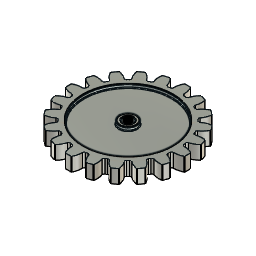
spur gear (Autodesk Fusion 360 design; units mm, degrees)
part number: 2025-09-15-00-14-42-283
Autodesk Fusion 360 part; units mm, degrees
sketch "Sketch1" plane through (0, 0, 0) normal (0, 0, 1) x (1, 0, 0)
  line L0 (0, 0) -> (0, 120) construction
  line L1 (0, 0) -> (120, 0) construction
  line L2 (7.5783, 72.1028) -> (12.464, 118.5873)
  line L3 (13.688, 86.4227) -> (18.0383, 113.8896)
  arc A0 (7.7182, 74.3498) -> (4.8497, 86.8626) centre (-18.7417, 74.8692) ccw
  arc A1 (4.0041, 87.4083) -> (-4.0041, 87.4083) centre (0, 0) ccw
  arc A2 (7.2846, 79.6676) -> (80, 0) centre (0, 0) ccw
  line L4 (11.3415, 71.6074) -> (0, 0)
  arc A3 (11.3415, 71.6074) -> (9.8771, 71.824) centre (0, 0) ccw
  arc A4 (7.7182, 74.3498) -> (9.8771, 71.824) centre (10.2177, 74.3007) ccw
  arc A5 (4.8497, 86.8626) -> (4.0041, 87.4083) centre (3.9583, 86.4094) ccw
  line L5 (-11.3415, 71.6074) -> (0, 0)
  arc A6 (-9.8771, 71.824) -> (-7.7182, 74.3498) centre (-10.2177, 74.3007) ccw
  arc A7 (-9.8771, 71.824) -> (-11.3415, 71.6074) centre (0, 0) ccw
  arc A8 (-4.8497, 86.8626) -> (-7.7182, 74.3498) centre (18.7417, 74.8692) ccw
  arc A9 (-4.0041, 87.4083) -> (-4.8497, 86.8626) centre (-3.9583, 86.4094) ccw
  arc A10 (-87.5, 0) -> (87.5, 0) centre (0, 0) ccw
  arc A11 (13.688, 86.4227) -> (-4.0041, 87.4083) centre (0, 0) ccw
  dimension "d1" = 160
  dimension "d2" = 175
  dimension "d3" = 145
  dimension "d5" = 6
  dimension "d6" = 9
  dimension "d7" = 2.5
  dimension "d8" = 1
  constraint coincident L0.start L1.start
  constraint concentric A1 A2
  constraint vertical L0
  constraint perpendicular L0 L1
  constraint tangent L2 A0
  constraint coincident L1 A10.end
  constraint coincident L1 A2.end
  constraint coincident A0 A2.start
  constraint coincident L2.start A3
  constraint coincident L2.start A0
  constraint tangent A3 A4
  constraint tangent A0 A4
  constraint tangent A0 A5
  constraint tangent A1 A5
  constraint symmetric L0 A0 A8
  constraint symmetric L0 A10.end A10.start
  constraint symmetric L0 A1 A10
  constraint symmetric L0 L4.start L5.start
  constraint symmetric L0 L1.start A1.centre
  constraint symmetric L0 A3 A7
  constraint symmetric L0 A3.end A6.start
  constraint symmetric L0 A0.start A6.end
  constraint symmetric L0 A4 A6
  constraint symmetric L0 A0.end A8.start
  constraint symmetric L0 A1.start A1.end
  constraint symmetric L0 A5 A9
  constraint concentric A10 A11
  measures "d1" diameter of A2
  measures "d2" diameter of A1
  measures "d3" diameter of A3
  measures "d5" angle of L0 L2
  measures "d6" angle of L0 L3
  measures "d7" radius of A4
  measures "d8" radius of A5
sketch "Sketch2" plane through (0, 0, 0) normal (0, 0, 1) x (1, 0, 0)
extrude "Extrude1" add sketch "Sketch1" along normal blind 20 contours A0 A2 L4 A3 A4 L5 A6 A7 A8 | A0 A1 A2 A5 A8 A9 A11 makes body 1
pattern_circular "C-Pattern1" count 20 over 360 about axis through (0, 0, 1.75) along (0, 0, 1) of bodies 1 makes body 2 at (-7.561, 47.7383, 6.6667) makes body 3 at (-28.1691, 38.7805, 0) makes body 4 at (-38.7742, 28.1777, 0) makes body 5 at (-45.5839, 14.8167, 0) makes body 6 at (-47.9315, 0.0054, 0) makes body 7 at (-45.5872, -14.8066, 0) makes body 8 at (-38.7805, -28.1691, 0) makes body 9 at (-28.1777, -38.7742, 0) makes body 10 at (-14.8167, -45.5839, 0) makes body 11 at (-0.0054, -47.9315, 0) makes body 12 at (14.8066, -45.5872, 0) makes body 13 at (28.1691, -38.7805, 0) makes body 14 at (38.7742, -28.1777, 0) makes body 15 at (45.5839, -14.8167, 0) makes body 16 at (47.9315, -0.0054, 0) makes body 17 at (45.5872, 14.8066, 0) makes body 18 at (38.7805, 28.1691, 0) makes body 19 at (28.1777, 38.7742, 0) makes body 20 at (7.561, 47.7383, 6.6667)
combine "Combine1" operation add target body 20 tool bodies 19 18 17 16 15 14 13 12 11 10 9 8 7 6 5 4 3 2 1
sketch "Sketch3" plane through (0, 0, 20) normal (0, 0, 1) x (-1, 0, 0)
  arc A0 (-30.3158, -68.3258) -> (-31.4544, -81.1126) centre (-5.3114, -76.9963) ccw
  arc A1 (-31.4544, -81.1126) -> (-30.8187, -81.8929) centre (-30.4665, -80.957) ccw
  arc A2 (-30.8187, -81.8929) -> (-23.2026, -84.3676) centre (0, 0) ccw
  arc A3 (-23.2026, -84.3676) -> (-22.2297, -84.1099) centre (-22.9374, -83.4034) ccw
  arc A4 (-22.2297, -84.1099) -> (-15.6349, -73.0959) centre (-40.9603, -65.4133) ccw
  arc A5 (-12.8011, -71.3609) -> (-15.6349, -73.0959) centre (-13.2426, -73.8216) ccw
  arc A6 (-12.8011, -71.3609) -> (-9.8771, -71.824) centre (0, 0) ccw
  arc A7 (-7.7182, -74.3498) -> (-9.8771, -71.824) centre (-10.2177, -74.3007) ccw
  arc A8 (-7.7182, -74.3498) -> (-4.8497, -86.8626) centre (18.7417, -74.8692) ccw
  arc A9 (-4.8497, -86.8626) -> (-4.0041, -87.4083) centre (-3.9583, -86.4094) ccw
  arc A10 (-4.0041, -87.4083) -> (4.0041, -87.4083) centre (0, 0) ccw
  arc A11 (4.0041, -87.4083) -> (4.8497, -86.8626) centre (3.9583, -86.4094) ccw
  arc A12 (4.8497, -86.8626) -> (7.7182, -74.3498) centre (-18.7417, -74.8692) ccw
  arc A13 (9.8771, -71.824) -> (7.7182, -74.3498) centre (10.2177, -74.3007) ccw
  arc A14 (9.8771, -71.824) -> (12.8011, -71.3609) centre (0, 0) ccw
  arc A15 (15.6349, -73.0959) -> (12.8011, -71.3609) centre (13.2426, -73.8216) ccw
  arc A16 (15.6349, -73.0959) -> (22.2297, -84.1099) centre (40.9603, -65.4133) ccw
  arc A17 (22.2297, -84.1099) -> (23.2026, -84.3676) centre (22.9374, -83.4034) ccw
  arc A18 (23.2026, -84.3676) -> (30.8187, -81.8929) centre (0, 0) ccw
  arc A19 (30.8187, -81.8929) -> (31.4544, -81.1126) centre (30.4665, -80.957) ccw
  arc A20 (31.4544, -81.1126) -> (30.3158, -68.3258) centre (5.3114, -76.9963) ccw
  arc A21 (31.5886, -65.2565) -> (30.3158, -68.3258) centre (32.6778, -67.5067) ccw
  arc A22 (31.5886, -65.2565) -> (34.2264, -63.9125) centre (0, 0) ccw
  arc A23 (37.4576, -64.6869) -> (34.2264, -63.9125) centre (35.4066, -66.1164) ccw
  arc A24 (37.4576, -64.6869) -> (47.133, -73.1239) centre (59.1694, -49.5543) ccw
  arc A25 (47.133, -73.1239) -> (48.138, -73.0684) centre (47.5878, -72.2333) ccw
  arc A26 (48.138, -73.0684) -> (54.6167, -68.3613) centre (0, 0) ccw
  arc A27 (54.6167, -68.3613) -> (54.98, -67.4227) centre (53.9925, -67.58) ccw
  arc A28 (54.98, -67.4227) -> (49.9459, -55.6136) centre (28.8446, -71.5866) ccw
  arc A29 (50.2079, -52.3012) -> (49.9459, -55.6136) centre (51.9392, -54.1047) ccw
  arc A30 (50.2079, -52.3012) -> (52.3012, -50.2079) centre (0, 0) ccw
  arc A31 (55.6136, -49.9459) -> (52.3012, -50.2079) centre (54.1047, -51.9392) ccw
  arc A32 (55.6136, -49.9459) -> (67.4227, -54.98) centre (71.5866, -28.8446) ccw
  arc A33 (67.4227, -54.98) -> (68.3613, -54.6167) centre (67.58, -53.9925) ccw
  arc A34 (68.3613, -54.6167) -> (73.0684, -48.138) centre (0, 0) ccw
  arc A35 (73.0684, -48.138) -> (73.1239, -47.133) centre (72.2333, -47.5878) ccw
  arc A36 (73.1239, -47.133) -> (64.6869, -37.4576) centre (49.5543, -59.1694) ccw
  arc A37 (63.9125, -34.2264) -> (64.6869, -37.4576) centre (66.1164, -35.4066) ccw
  arc A38 (63.9125, -34.2264) -> (65.2565, -31.5886) centre (0, 0) ccw
  arc A39 (68.3258, -30.3158) -> (65.2565, -31.5886) centre (67.5067, -32.6778) ccw
  arc A40 (68.3258, -30.3158) -> (81.1126, -31.4544) centre (76.9963, -5.3114) ccw
  arc A41 (81.1126, -31.4544) -> (81.8929, -30.8187) centre (80.957, -30.4665) ccw
  arc A42 (81.8929, -30.8187) -> (84.3676, -23.2026) centre (0, 0) ccw
  arc A43 (84.3676, -23.2026) -> (84.1099, -22.2297) centre (83.4034, -22.9374) ccw
  arc A44 (84.1099, -22.2297) -> (73.0959, -15.6349) centre (65.4133, -40.9603) ccw
  arc A45 (71.3609, -12.8011) -> (73.0959, -15.6349) centre (73.8216, -13.2426) ccw
  arc A46 (71.3609, -12.8011) -> (71.824, -9.8771) centre (0, 0) ccw
  arc A47 (74.3498, -7.7182) -> (71.824, -9.8771) centre (74.3007, -10.2177) ccw
  arc A48 (74.3498, -7.7182) -> (86.8626, -4.8497) centre (74.8692, 18.7417) ccw
  arc A49 (86.8626, -4.8497) -> (87.4083, -4.0041) centre (86.4094, -3.9583) ccw
  arc A50 (87.4083, -4.0041) -> (87.4083, 4.0041) centre (0, 0) ccw
  arc A51 (87.4083, 4.0041) -> (86.8626, 4.8497) centre (86.4094, 3.9583) ccw
  arc A52 (86.8626, 4.8497) -> (74.3498, 7.7182) centre (74.8692, -18.7417) ccw
  arc A53 (71.824, 9.8771) -> (74.3498, 7.7182) centre (74.3007, 10.2177) ccw
  arc A54 (71.824, 9.8771) -> (71.3609, 12.8011) centre (0, 0) ccw
  arc A55 (73.0959, 15.6349) -> (71.3609, 12.8011) centre (73.8216, 13.2426) ccw
  arc A56 (73.0959, 15.6349) -> (84.1099, 22.2297) centre (65.4133, 40.9603) ccw
  arc A57 (84.1099, 22.2297) -> (84.3676, 23.2026) centre (83.4034, 22.9374) ccw
  arc A58 (84.3676, 23.2026) -> (81.8929, 30.8187) centre (0, 0) ccw
  arc A59 (81.8929, 30.8187) -> (81.1126, 31.4544) centre (80.957, 30.4665) ccw
  arc A60 (81.1126, 31.4544) -> (68.3258, 30.3158) centre (76.9963, 5.3114) ccw
  arc A61 (65.2565, 31.5886) -> (68.3258, 30.3158) centre (67.5067, 32.6778) ccw
  arc A62 (65.2565, 31.5886) -> (63.9125, 34.2264) centre (0, 0) ccw
  arc A63 (64.6869, 37.4576) -> (63.9125, 34.2264) centre (66.1164, 35.4066) ccw
  arc A64 (64.6869, 37.4576) -> (73.1239, 47.133) centre (49.5543, 59.1694) ccw
  arc A65 (73.1239, 47.133) -> (73.0684, 48.138) centre (72.2333, 47.5878) ccw
  arc A66 (73.0684, 48.138) -> (68.3613, 54.6167) centre (0, 0) ccw
  arc A67 (68.3613, 54.6167) -> (67.4227, 54.98) centre (67.58, 53.9925) ccw
  arc A68 (67.4227, 54.98) -> (55.6136, 49.9459) centre (71.5866, 28.8446) ccw
  arc A69 (52.3012, 50.2079) -> (55.6136, 49.9459) centre (54.1047, 51.9392) ccw
  arc A70 (52.3012, 50.2079) -> (50.2079, 52.3012) centre (0, 0) ccw
  arc A71 (49.9459, 55.6136) -> (50.2079, 52.3012) centre (51.9392, 54.1047) ccw
  arc A72 (49.9459, 55.6136) -> (54.98, 67.4227) centre (28.8446, 71.5866) ccw
  arc A73 (54.98, 67.4227) -> (54.6167, 68.3613) centre (53.9925, 67.58) ccw
  arc A74 (54.6167, 68.3613) -> (48.138, 73.0684) centre (0, 0) ccw
  arc A75 (48.138, 73.0684) -> (47.133, 73.1239) centre (47.5878, 72.2333) ccw
  arc A76 (47.133, 73.1239) -> (37.4576, 64.6869) centre (59.1694, 49.5543) ccw
  arc A77 (34.2264, 63.9125) -> (37.4576, 64.6869) centre (35.4066, 66.1164) ccw
  arc A78 (34.2264, 63.9125) -> (31.5886, 65.2565) centre (0, 0) ccw
  arc A79 (30.3158, 68.3258) -> (31.5886, 65.2565) centre (32.6778, 67.5067) ccw
  arc A80 (30.3158, 68.3258) -> (31.4544, 81.1126) centre (5.3114, 76.9963) ccw
  arc A81 (31.4544, 81.1126) -> (30.8187, 81.8929) centre (30.4665, 80.957) ccw
  arc A82 (30.8187, 81.8929) -> (23.2026, 84.3676) centre (0, 0) ccw
  arc A83 (23.2026, 84.3676) -> (22.2297, 84.1099) centre (22.9374, 83.4034) ccw
  arc A84 (22.2297, 84.1099) -> (15.6349, 73.0959) centre (40.9603, 65.4133) ccw
  arc A85 (12.8011, 71.3609) -> (15.6349, 73.0959) centre (13.2426, 73.8216) ccw
  arc A86 (12.8011, 71.3609) -> (9.8771, 71.824) centre (0, 0) ccw
  arc A87 (7.7182, 74.3498) -> (9.8771, 71.824) centre (10.2177, 74.3007) ccw
  arc A88 (7.7182, 74.3498) -> (4.8497, 86.8626) centre (-18.7417, 74.8692) ccw
  arc A89 (4.8497, 86.8626) -> (4.0041, 87.4083) centre (3.9583, 86.4094) ccw
  arc A90 (4.0041, 87.4083) -> (-4.0041, 87.4083) centre (0, 0) ccw
  arc A91 (-4.0041, 87.4083) -> (-4.8497, 86.8626) centre (-3.9583, 86.4094) ccw
  arc A92 (-4.8497, 86.8626) -> (-7.7182, 74.3498) centre (18.7417, 74.8692) ccw
  arc A93 (-9.8771, 71.824) -> (-7.7182, 74.3498) centre (-10.2177, 74.3007) ccw
  arc A94 (-9.8771, 71.824) -> (-12.8011, 71.3609) centre (0, 0) ccw
  arc A95 (-15.6349, 73.0959) -> (-12.8011, 71.3609) centre (-13.2426, 73.8216) ccw
  arc A96 (-15.6349, 73.0959) -> (-22.2297, 84.1099) centre (-40.9603, 65.4133) ccw
  arc A97 (-22.2297, 84.1099) -> (-23.2026, 84.3676) centre (-22.9374, 83.4034) ccw
  arc A98 (-23.2026, 84.3676) -> (-30.8187, 81.8929) centre (0, 0) ccw
  arc A99 (-30.8187, 81.8929) -> (-31.4544, 81.1126) centre (-30.4665, 80.957) ccw
  arc A100 (-31.4544, 81.1126) -> (-30.3158, 68.3258) centre (-5.3114, 76.9963) ccw
  arc A101 (-31.5886, 65.2565) -> (-30.3158, 68.3258) centre (-32.6778, 67.5067) ccw
  arc A102 (-31.5886, 65.2565) -> (-34.2264, 63.9125) centre (0, 0) ccw
  arc A103 (-37.4576, 64.6869) -> (-34.2264, 63.9125) centre (-35.4066, 66.1164) ccw
  arc A104 (-37.4576, 64.6869) -> (-47.133, 73.1239) centre (-59.1694, 49.5543) ccw
  arc A105 (-47.133, 73.1239) -> (-48.138, 73.0684) centre (-47.5878, 72.2333) ccw
  arc A106 (-48.138, 73.0684) -> (-54.6167, 68.3613) centre (0, 0) ccw
  arc A107 (-54.6167, 68.3613) -> (-54.98, 67.4227) centre (-53.9925, 67.58) ccw
  arc A108 (-54.98, 67.4227) -> (-49.9459, 55.6136) centre (-28.8446, 71.5866) ccw
  arc A109 (-50.2079, 52.3012) -> (-49.9459, 55.6136) centre (-51.9392, 54.1047) ccw
  arc A110 (-50.2079, 52.3012) -> (-52.3012, 50.2079) centre (0, 0) ccw
  arc A111 (-55.6136, 49.9459) -> (-52.3012, 50.2079) centre (-54.1047, 51.9392) ccw
  arc A112 (-55.6136, 49.9459) -> (-67.4227, 54.98) centre (-71.5866, 28.8446) ccw
  arc A113 (-67.4227, 54.98) -> (-68.3613, 54.6167) centre (-67.58, 53.9925) ccw
  arc A114 (-68.3613, 54.6167) -> (-73.0684, 48.138) centre (0, 0) ccw
  arc A115 (-73.0684, 48.138) -> (-73.1239, 47.133) centre (-72.2333, 47.5878) ccw
  arc A116 (-73.1239, 47.133) -> (-64.6869, 37.4576) centre (-49.5543, 59.1694) ccw
  arc A117 (-63.9125, 34.2264) -> (-64.6869, 37.4576) centre (-66.1164, 35.4066) ccw
  arc A118 (-63.9125, 34.2264) -> (-65.2565, 31.5886) centre (0, 0) ccw
  arc A119 (-68.3258, 30.3158) -> (-65.2565, 31.5886) centre (-67.5067, 32.6778) ccw
  arc A120 (-68.3258, 30.3158) -> (-81.1126, 31.4544) centre (-76.9963, 5.3114) ccw
  arc A121 (-81.1126, 31.4544) -> (-81.8929, 30.8187) centre (-80.957, 30.4665) ccw
  arc A122 (-81.8929, 30.8187) -> (-84.3676, 23.2026) centre (0, 0) ccw
  arc A123 (-84.3676, 23.2026) -> (-84.1099, 22.2297) centre (-83.4034, 22.9374) ccw
  arc A124 (-84.1099, 22.2297) -> (-73.0959, 15.6349) centre (-65.4133, 40.9603) ccw
  arc A125 (-71.3609, 12.8011) -> (-73.0959, 15.6349) centre (-73.8216, 13.2426) ccw
  arc A126 (-71.3609, 12.8011) -> (-71.824, 9.8771) centre (0, 0) ccw
  arc A127 (-74.3498, 7.7182) -> (-71.824, 9.8771) centre (-74.3007, 10.2177) ccw
  arc A128 (-74.3498, 7.7182) -> (-86.8626, 4.8497) centre (-74.8692, -18.7417) ccw
  arc A129 (-86.8626, 4.8497) -> (-87.4083, 4.0041) centre (-86.4094, 3.9583) ccw
  arc A130 (-87.4083, 4.0041) -> (-87.4083, -4.0041) centre (0, 0) ccw
  arc A131 (-87.4083, -4.0041) -> (-86.8626, -4.8497) centre (-86.4094, -3.9583) ccw
  arc A132 (-86.8626, -4.8497) -> (-74.3498, -7.7182) centre (-74.8692, 18.7417) ccw
  arc A133 (-71.824, -9.8771) -> (-74.3498, -7.7182) centre (-74.3007, -10.2177) ccw
  arc A134 (-71.824, -9.8771) -> (-71.3609, -12.8011) centre (0, 0) ccw
  arc A135 (-73.0959, -15.6349) -> (-71.3609, -12.8011) centre (-73.8216, -13.2426) ccw
  arc A136 (-73.0959, -15.6349) -> (-84.1099, -22.2297) centre (-65.4133, -40.9603) ccw
  arc A137 (-84.1099, -22.2297) -> (-84.3676, -23.2026) centre (-83.4034, -22.9374) ccw
  arc A138 (-84.3676, -23.2026) -> (-81.8929, -30.8187) centre (0, 0) ccw
  arc A139 (-81.8929, -30.8187) -> (-81.1126, -31.4544) centre (-80.957, -30.4665) ccw
  arc A140 (-81.1126, -31.4544) -> (-68.3258, -30.3158) centre (-76.9963, -5.3114) ccw
  arc A141 (-65.2565, -31.5886) -> (-68.3258, -30.3158) centre (-67.5067, -32.6778) ccw
  arc A142 (-65.2565, -31.5886) -> (-63.9125, -34.2264) centre (0, 0) ccw
  arc A143 (-64.6869, -37.4576) -> (-63.9125, -34.2264) centre (-66.1164, -35.4066) ccw
  arc A144 (-64.6869, -37.4576) -> (-73.1239, -47.133) centre (-49.5543, -59.1694) ccw
  arc A145 (-73.1239, -47.133) -> (-73.0684, -48.138) centre (-72.2333, -47.5878) ccw
  arc A146 (-73.0684, -48.138) -> (-68.3613, -54.6167) centre (0, 0) ccw
  arc A147 (-68.3613, -54.6167) -> (-67.4227, -54.98) centre (-67.58, -53.9925) ccw
  arc A148 (-67.4227, -54.98) -> (-55.6136, -49.9459) centre (-71.5866, -28.8446) ccw
  arc A149 (-52.3012, -50.2079) -> (-55.6136, -49.9459) centre (-54.1047, -51.9392) ccw
  arc A150 (-52.3012, -50.2079) -> (-50.2079, -52.3012) centre (0, 0) ccw
  arc A151 (-49.9459, -55.6136) -> (-50.2079, -52.3012) centre (-51.9392, -54.1047) ccw
  arc A152 (-49.9459, -55.6136) -> (-54.98, -67.4227) centre (-28.8446, -71.5866) ccw
  arc A153 (-54.98, -67.4227) -> (-54.6167, -68.3613) centre (-53.9925, -67.58) ccw
  arc A154 (-54.6167, -68.3613) -> (-48.138, -73.0684) centre (0, 0) ccw
  arc A155 (-48.138, -73.0684) -> (-47.133, -73.1239) centre (-47.5878, -72.2333) ccw
  arc A156 (-47.133, -73.1239) -> (-37.4576, -64.6869) centre (-59.1694, -49.5543) ccw
  arc A157 (-34.2264, -63.9125) -> (-37.4576, -64.6869) centre (-35.4066, -66.1164) ccw
  arc A158 (-34.2264, -63.9125) -> (-31.5886, -65.2565) centre (0, 0) ccw
  arc A159 (-30.3158, -68.3258) -> (-31.5886, -65.2565) centre (-32.6778, -67.5067) ccw
  circle A160 centre (0, 0) radius 65
  circle A161 centre (0, 0) radius 7.5
  circle A162 centre (0, 0) radius 12.5
  dimension "d13" = 130
  dimension "d14" = 15
  dimension "d15" = 25
  constraint coincident A2.centre A6.centre
  constraint concentric A161 A162
  measures "d13" diameter of A160
  measures "d14" diameter of A161
  measures "d15" diameter of A162
extrude "Extrude2" cut sketch "Sketch3" against normal blind 5 contours A160 bodies 20
extrude "Extrude3" cut sketch "Sketch3" against normal blind 110 contours A161 bodies 20
fillet "Fillet1" radius 1 3 edges at (60.6013, -23.505, 20) (11.6541, 4.5202, 20) (6.9925, -2.7121, 20) on bodies 20
fillet "Fillet2" radius 1 2 edges at (60.6013, -23.505, 15) (11.6541, 4.5202, 15) on bodies 20
